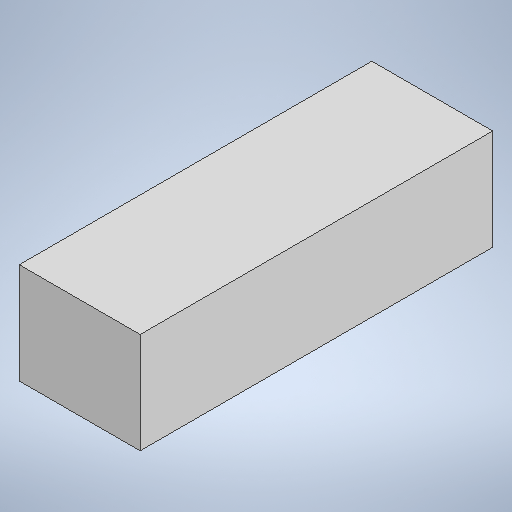
# Autodesk Inventor part: Lipo Battery 9500mAh 22.2V
Saved by Autodesk Inventor 2025.1 (Build 291241000, 241)
## iProperties
Created: 2025-04-08
Part Number: Lipo Battery 9500mAh 22.2V
Material: Типовые
Document SubType Name: Modeling
Designer: Root
Density: 1 g/cm^3
Appearance: По умолчанию
Author: Root
Autodesk Inventor part; units mm, degrees
ref_plane "YZ Plane" through (0, 0, 0) normal (1, 0, 0) x (0, 1, 0)
ref_plane "XZ Plane" through (0, 0, 0) normal (0, 1, 0) x (-1, 0, 0)
ref_plane "XY Plane" through (0, 0, 0) normal (0, 0, 1) x (1, 0, 0)
sketch "Эскиз1" plane through (0, 0, 0) normal (0, 1, 0) x (-1, 0, 0)
  line L0 (-30, -87.5) -> (30, -87.5)
  line L1 (30, -87.5) -> (30, 87.5)
  line L2 (30, 87.5) -> (-30, 87.5)
  line L3 (-30, 87.5) -> (-30, -87.5)
  line L4 (-30, -87.5) -> (30, 87.5) construction
  line L5 (30, -87.5) -> (-30, 87.5) construction
  point P0 (0, 0)
  dimension "d0" = 60
  dimension "d1" = 175
  constraints: 12 end point, 2 midpoint, 2 parallel, 1 horizontal, 1 perpendicular
  measures "d0" distance of L2.end L1.end
  measures "d1" distance of L1.end L0.end
extrude "Выдавливание1" add sketch "Эскиз1" along normal mid plane 50
